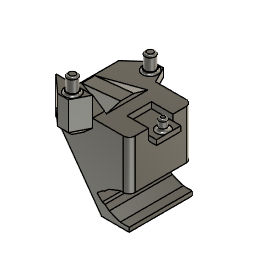
whiteboard v7 (Autodesk Fusion 360 archive; units mm, degrees)
design "Centre_pulley_mount"
Autodesk Fusion 360 part; units mm, degrees
sketch "Sketch1" plane through (0, 0, 0) normal (0, 1, 0) x (1, 0, 0)
  line L0 (36.78, 0) -> (0, 0)
  line L1 (0, 0) -> (0, -40.3)
  line L2 (0, -40.3) -> (6.2098, -40.3)
  line L3 (15.9457, -40.3) -> (36.78, -40.3)
  line L4 (18.4769, -2.1208) -> (18.4964, -2.1208)
  line L5 (36.78, -40.3) -> (36.78, -15.7708)
  line L6 (36.78, -2.0947) -> (36.78, 0)
  line L7 (6.2098, -40.3) -> (15.9457, -40.3)
  line L8 (26.7841, -13.675) -> (24.3642, -11.6584)
  line L9 (32.31, -15.7708) -> (26.7841, -13.675)
  line L10 (36.78, -15.7708) -> (32.31, -15.7708)
  line L11 (36.7605, -2.1208) -> (32.2906, -2.1335)
  line L12 (32.2906, -2.1335) -> (26.7706, -4.2451)
  line L13 (26.7706, -4.2451) -> (24.643, -6.0284)
  line L14 (36.7605, -2.1208) -> (36.78, -2.1208)
  line L15 (36.78, -2.1208) -> (36.78, -2.0947)
  line L16 (24.3642, -11.6584) -> (23.2561, -11.1913)
  line L17 (23.2561, -11.1913) -> (20.661, -9.0288)
  line L18 (24.643, -6.0284) -> (23.3467, -6.4358)
  line L19 (23.3467, -6.4358) -> (20.661, -9.0288)
  point P0 (18.4964, -8.9458)
  point P1 (18.4964, -8.9458)
  point P2 (36.6848, -8.6861)
  point P3 (36.6848, -8.6861)
  point P4 (36.78, -8.9458)
  point P5 (36.78, -8.9458)
  dimension "d19" = 40.3
  dimension "d21" = 36.78
  dimension "d31" = 13.65
  dimension "d32" = 4.47
  dimension "d33" = 159.23
  dimension "d34" = 160.964
  dimension "d36" = 5.91
  dimension "d37" = 3.15
  constraint horizontal L2
  constraint vertical L5
  constraint horizontal L0
  constraint vertical L1
  constraint collinear L2 L3
  constraint coincident P1 P0
  constraint coincident L0.end L1.start
  constraint collinear L5 L6
  constraint coincident L4 L6.start
  constraint parallel L3 L7
  constraint coincident P3 P2
  constraint coincident P5 P4
  constraint coincident L5.end L10.start
  constraint parallel L6 L15
  constraint parallel L8 L17
  measures "d19" distance of L1.end L0.end
  measures "d21" distance of L1 L5
  measures "d31" distance of L14.end L5.end
  measures "d32" distance of L9.start L5.end
  measures "d33" angle of L9 L10
  measures "d34" angle of L8 L9
  measures "d36" distance of L8.start L9.start
  measures "d37" distance of L8.start L8.end
extrude "Extrude1" add sketch "Sketch1" along normal blind 31.6
sketch "Sketch2" plane through (0, 0, 40.3) normal (0, 0, 1) x (-1, 0, 0)
  line L0 (0, 0) -> (-36.78, 0)
  line L1 (-36.78, 0) -> (-36.78, -31.6)
  line L2 (-36.78, -31.6) -> (0, -31.6)
  line L3 (0, -31.6) -> (0, 0)
  line L4 (-26, -21.9) -> (-36.78, -21.9)
  line L5 (-36.78, -21.9) -> (-36.78, -9.7)
  line L6 (-36.78, -9.7) -> (-26, -9.7)
  line L7 (-26, -9.7) -> (-26, -21.9)
  point P0 (-36.78, -15.8)
  point P1 (-36.78, -15.8)
  dimension "d42" = 12.2
  dimension "d43" = 10.78
  constraint horizontal L4
  constraint vertical L5
  constraint horizontal L6
  constraint vertical L7
  constraint coincident L1 L5.end
  constraint midpoint L5 P1
  constraint midpoint L1 P1
  constraint coincident P1 P0
  measures "d42" distance of L4.start L6.end
  measures "d43" distance of L4.start L4.end
extrude "Extrude2" cut sketch "Sketch2" against normal blind 2.5 contours L1 L4 L5 L6 L7
sketch "Sketch3" plane through (36.78, 0, 0) normal (1, 0, 0) x (0, 1, 0)
  line L0 (9.7, 37.8) -> (9.7, 40.3)
  line L1 (9.7, 40.3) -> (0, 40.3)
  line L2 (0, 40.3) -> (0, 15.7708)
  line L3 (0, 15.7708) -> (31.6, 15.7708)
  line L4 (31.6, 15.7708) -> (31.6, 40.3)
  line L5 (31.6, 40.3) -> (21.9, 40.3)
  line L6 (21.9, 40.3) -> (21.9, 37.8)
  line L7 (21.9, 37.8) -> (9.7, 37.8)
  line L8 (9.7, 37.8) -> (21.9, 37.8)
  line L9 (21.9, 37.8) -> (21.9, 35.8)
  line L10 (21.9, 35.8) -> (9.7, 35.8)
  line L11 (9.7, 35.8) -> (9.7, 37.8)
  dimension "d46" = 2
  constraint horizontal L8
  constraint vertical L9
  constraint horizontal L10
  constraint vertical L11
  constraint coincident L0.start L7.end
  constraint collinear L6 L9
  measures "d46" distance of L0.start L10.end
extrude "Extrude3" add sketch "Sketch3" along normal blind 3 contours L7 L8 L9 L10 L11
sketch "Sketch4" plane through (0, 0, 37.8) normal (0, 0, 1) x (-1, 0, 0)
  line L0 (-26, -9.7) -> (-36.78, -9.7)
  line L1 (-36.78, -9.7) -> (-39.78, -9.7)
  line L2 (-39.78, -9.7) -> (-39.78, -21.9)
  line L3 (-39.78, -21.9) -> (-36.78, -21.9)
  line L4 (-36.78, -21.9) -> (-26, -21.9)
  line L5 (-26, -21.9) -> (-26, -9.7)
  circle A0 centre (-37.9, -15.8) radius 1.9
  point P0 (-39.78, -15.8)
  dimension "d49" = 3.8
  dimension "d50" = 11.9
  constraint midpoint L2 P0
  constraint horizontal A0.centre P0
  measures "d49" diameter of A0
  measures "d50" distance of L5 A0.centre
extrude "Extrude4" add 1 faces at (39.78, 13.7667, 36.4667) along direction (1, 0, 0) blind 0.5
extrude "Extrude5" add sketch "Sketch4" along normal blind 5 contours L2 A0 | L2 A0
sketch "Sketch5" plane through (0, 0, 0) normal (0, -1, 0) x (1, 0, 0)
  line L0 (36.78, 2.1208) -> (36.7605, 2.1208)
  line L1 (36.7605, 2.1208) -> (32.2906, 2.1335)
  line L2 (32.2906, 2.1335) -> (26.7706, 4.2451)
  line L3 (26.7706, 4.2451) -> (24.643, 6.0284)
  line L4 (24.3642, 11.6584) -> (26.7841, 13.675)
  line L5 (26.7841, 13.675) -> (32.31, 15.7708)
  line L6 (32.31, 15.7708) -> (36.78, 15.7708)
  line L7 (36.78, 15.7708) -> (36.78, 40.3)
  line L8 (36.78, 40.3) -> (0, 40.3)
  line L9 (0, 40.3) -> (0, 0)
  line L10 (0, 0) -> (36.78, 0)
  line L11 (36.78, 0) -> (36.78, 2.1208)
  line L12 (0, 40.3) -> (18.39, 40.3)
  line L13 (18.39, 40.3) -> (18.39, 27.8397)
  line L14 (18.39, 27.8397) -> (0, 27.8397)
  line L15 (0, 27.8397) -> (0, 40.3)
  line L16 (24.643, 6.0284) -> (23.3467, 6.4358)
  line L17 (23.3467, 6.4358) -> (20.661, 9.0288)
  line L18 (20.661, 9.0288) -> (23.2561, 11.1913)
  line L19 (23.2561, 11.1913) -> (24.3642, 11.6584)
  point P0 (18.39, 40.3)
  constraint horizontal L12
  constraint vertical L13
  constraint horizontal L14
  constraint vertical L15
  constraint coincident L8.end L9.start
  constraint midpoint L8 P0
  constraint coincident P0 L12.end
extrude "Extrude6" add sketch "Sketch5" along normal blind 10 contours L8 L9 L12 L13 L14 L15
sketch "Sketch6" plane through (0, 0, 40.3) normal (0, 0, 1) x (-1, 0, 0)
  line L0 (-36.78, -9.7) -> (-26, -9.7)
  line L1 (-26, -9.7) -> (-26, -21.9)
  line L2 (-26, -21.9) -> (-36.78, -21.9)
  line L3 (-36.78, -21.9) -> (-36.78, -31.6)
  line L4 (-36.78, -31.6) -> (0, -31.6)
  line L5 (0, -31.6) -> (0, 10)
  line L6 (0, 10) -> (-18.39, 10)
  line L7 (-18.39, 10) -> (-18.39, 0)
  line L8 (-18.39, 0) -> (-36.78, 0)
  line L9 (-36.78, 0) -> (-36.78, -9.7)
  circle A0 centre (-12, 3.7) radius 2.5
  line L10 (-26, -15.8) -> (0, -15.8) construction
  circle A1 centre (-12, -35.3) radius 2.5
  dimension "d57" = 5
  dimension "d58" = 12
  dimension "d59" = 19.5
  dimension "d69" = 5
  constraint midpoint L1 L10.start
  constraint coincident L5 L10.end
  constraint perpendicular L5 L10
  constraint symmetric A0 L10 A1
  measures "d57" diameter of A0
  measures "d58" distance of L5 A0.centre
  measures "d59" distance of A0.centre L10
  measures "d69" diameter of A1
extrude "Extrude7" cut 1 faces at (6.13, -10, 36.1466) along direction (0, 1, 0) blind 2
chamfer "Chamfer1" distance 8 distance2 4 1 edges at (18.39, -8, 34.0698) measured on face at (18.39, -2.6667, 36.1466)
chamfer "Chamfer2" distance 8 distance2 9 1 edges at (0, -8, 34.0698) measured on face at (0, 21.0667, 22.7132)
chamfer "Chamfer3" distance 4 distance2 4 3 edges at (4.5, -4, 27.8397) (11.695, -8, 27.8397) (16.39, -4, 27.8397) measured on face at (6, -5.3333, 36.1466) measured on face at (9.13, -2.6667, 27.8397) measured on face at (17.0569, -2.6677, 36.1466)
sketch "Sketch7" plane through (0, 31.6, 0) normal (0, 1, 0) x (-1, 0, 0)
  line L0 (-36.7605, 2.1208) -> (-36.78, 2.1208)
  line L1 (-36.78, 2.1208) -> (-36.78, 0)
  line L2 (-36.78, 0) -> (0, 0)
  line L3 (0, 0) -> (0, 40.3)
  line L4 (0, 40.3) -> (-36.78, 40.3)
  line L5 (-36.78, 40.3) -> (-36.78, 15.7708)
  line L6 (-36.78, 15.7708) -> (-32.31, 15.7708)
  line L7 (-32.31, 15.7708) -> (-26.7841, 13.675)
  line L8 (-26.7841, 13.675) -> (-24.3642, 11.6584)
  line L9 (-24.643, 6.0284) -> (-26.7706, 4.2451)
  line L10 (-26.7706, 4.2451) -> (-32.2906, 2.1335)
  line L11 (-32.2906, 2.1335) -> (-36.7605, 2.1208)
  line L12 (0, 40.3) -> (-18.39, 40.3)
  line L13 (-18.39, 40.3) -> (-18.39, 32.3)
  line L14 (-18.39, 32.3) -> (0, 32.3)
  line L15 (0, 32.3) -> (0, 40.3)
  line L16 (-24.3642, 11.6584) -> (-23.2561, 11.1913)
  line L17 (-23.2561, 11.1913) -> (-20.661, 9.0288)
  line L18 (-20.661, 9.0288) -> (-23.3467, 6.4358)
  line L19 (-23.3467, 6.4358) -> (-24.643, 6.0284)
  point P0 (-18.39, 40.3)
  dimension "d68" = 8
  constraint horizontal L12
  constraint vertical L13
  constraint horizontal L14
  constraint vertical L15
  constraint coincident L3.end L4.start
  constraint midpoint L4 P0
  constraint coincident P0 L12.end
  measures "d68" distance of P0 L13.end
extrude "Extrude8" add sketch "Sketch7" along normal blind 8 contours L3 L4 L12 L13 L14 L15
chamfer "Chamfer4" distance 4 distance2 8 1 edges at (18.39, 39.6, 36.3) measured on face at (12.26, 39.6, 37.6333)
chamfer "Chamfer5" distance 9 distance2 8 1 edges at (0, 39.6, 36.3) measured on face at (4.7969, 39.6, 34.9667)
chamfer "Chamfer6" distance 4 distance2 4 3 edges at (11.695, 39.6, 32.3) (4.5, 35.6, 32.3) (16.39, 35.6, 32.3) measured on face at (12.5939, 39.6, 34.9667) measured on face at (6, 36.9333, 37.6333) measured on face at (17.0569, 34.2677, 37.6333)
extrude "Extrude9" add sketch "Sketch6" along normal blind 8 contours A0 | A1
sketch "Sketch8" plane through (0, 0, 40.3) normal (0, 0, 1) x (-1, 0, 0)
  circle A0 centre (-12, -35.3) radius 2.5
  circle A1 centre (-12, 3.7) radius 2.5
  line L0 (-9, -39.6) -> (0, -31.6)
  line L1 (0, -31.6) -> (0, 0)
  line L2 (0, 0) -> (-9, 8)
  line L3 (-9, 8) -> (-14.39, 8)
  line L4 (-14.39, 8) -> (-18.39, 0)
  line L5 (-18.39, 0) -> (-36.78, 0)
  line L6 (-36.78, 0) -> (-36.78, -9.7)
  line L7 (-36.78, -9.7) -> (-26, -9.7)
  line L8 (-26, -9.7) -> (-26, -21.9)
  line L9 (-26, -21.9) -> (-36.78, -21.9)
  line L10 (-36.78, -21.9) -> (-36.78, -31.6)
  line L11 (-36.78, -31.6) -> (-18.39, -31.6)
  line L12 (-18.39, -31.6) -> (-14.39, -39.6)
  line L13 (-14.39, -39.6) -> (-9, -39.6)
  circle A2 centre (-12, -35.3) radius 2.5
  circle A3 centre (-12, -35.3) radius 2.875
  dimension "d80" = 5.75
  constraint concentric A0 A2
  constraint concentric A2 A3
  measures "d80" diameter of A3
extrude "Extrude10" add sketch "Sketch8" along normal blind 1 contours A3
chamfer "Chamfer7" distance 23 distance2 32 1 edges at (0, 15.8, 0) measured on face at (24.52, 21.0667, 0)
fillet "Fillet1" radius 3 1 edges at (36.78, 0, 28.0354)
fillet "Fillet2" radius 3 1 edges at (36.78, 31.6, 28.0354)
fillet "Fillet3" radius 1 1 edges at (14.3308, 36.204, 48.3)
fillet "Fillet4" radius 1 1 edges at (39.6714, 16.4871, 42.8)
sketch "Sketch9" plane through (0, 0, 40.3) normal (0, 0, 1) x (-1, 0, 0)
  circle A0 centre (-12, -35.3) radius 2.875
  circle A1 centre (-12, 3.7) radius 2.5
  arc A2 (-36.78, -28.6) -> (-33.78, -31.6) centre (-33.78, -28.6) ccw
  line L0 (-33.78, -31.6) -> (-18.39, -31.6)
  line L1 (-18.39, -31.6) -> (-14.39, -39.6)
  line L2 (-14.39, -39.6) -> (-9, -39.6)
  line L3 (-9, -39.6) -> (0, -31.6)
  line L4 (0, -31.6) -> (0, 0)
  line L5 (0, 0) -> (-9, 8)
  line L6 (-9, 8) -> (-14.39, 8)
  line L7 (-14.39, 8) -> (-18.39, 0)
  line L8 (-18.39, 0) -> (-33.78, 0)
  arc A3 (-33.78, 0) -> (-36.78, -3) centre (-33.78, -3) ccw
  line L9 (-36.78, -3) -> (-36.78, -9.7)
  line L10 (-36.78, -9.7) -> (-26, -9.7)
  line L11 (-26, -9.7) -> (-26, -21.9)
  line L12 (-26, -21.9) -> (-36.78, -21.9)
  line L13 (-36.78, -21.9) -> (-36.78, -28.6)
  circle A4 centre (-12, 3.7) radius 2.5
  circle A5 centre (-12, 3.7) radius 2.875
  dimension "d93" = 5.75
  constraint concentric A1 A4
  constraint concentric A4 A5
  measures "d93" diameter of A5
extrude "Extrude11" add sketch "Sketch9" along normal blind 11 contours A5
extrude "Extrude12" add 1 faces at (11.2086, -2.7962, 48.3) along direction (0, 0, 1) blind 11
extrude "Extrude13" cut 1 faces at (11.2086, -2.7962, 59.3) along direction (0, 0, -1) blind 1
fillet "Fillet5" radius 1 1 edges at (14.3308, -4.604, 58.3)
sketch "Sketch10" plane through (0, 0, 0) normal (-1, 0, 0) x (0, -1, 0)
  line L0 (-31.6, 32) -> (0, 32)
  line L1 (0, 32) -> (0, 40.3)
  line L2 (0, 40.3) -> (-31.6, 40.3)
  line L3 (-31.6, 40.3) -> (-31.6, 36.3)
  line L4 (-31.6, 36.3) -> (-31.6, 32)
  line L5 (0, 32) -> (8.3989, 32)
  line L6 (8.3989, 32) -> (8.3989, 27.6433)
  line L7 (8.3989, 27.6433) -> (0, 27.6433)
  line L8 (0, 27.6433) -> (0, 32)
  constraint horizontal L5
  constraint vertical L6
  constraint horizontal L7
  constraint vertical L8
  constraint coincident L0.end L1.start
extrude "Extrude14" cut sketch "Sketch10" against normal blind 22 contours L5 L6 L7 L8
chamfer "Chamfer8" distance 4 distance2 4 3 edges at (4.5, -4, 32) (11.695, -8, 32) (16.39, -4, 32) measured on face at (3, -2.6667, 37.5333) measured on face at (12.5939, -8, 34.7667) measured on face at (15.7239, -5.3339, 37.5333)
sketch "Sketch11" plane through (0, 0, 40.3) normal (0, 0, 1) x (-1, 0, 0)
  circle A0 centre (-12, -35.3) radius 2.875
  circle A1 centre (-12, 3.7) radius 2.875
  line L0 (-0.5, -26.1) -> (-20, -26.1)
  line L1 (-20, -26.1) -> (-20, -5.5)
  line L2 (-20, -5.5) -> (-0.5, -5.5)
  line L3 (-0.5, -5.5) -> (-0.5, -26.1)
  line L4 (-26, -10.2) -> (-26, -21.9)
  arc A2 (-36.78, -28.6) -> (-33.78, -31.6) centre (-33.78, -28.6) ccw
  line L5 (-33.78, -31.6) -> (-18.39, -31.6)
  line L6 (-18.39, -31.6) -> (-14.39, -39.6)
  line L7 (-14.39, -39.6) -> (-9, -39.6)
  line L8 (-9, -39.6) -> (0, -31.6)
  line L9 (0, -31.6) -> (0, 0)
  line L10 (0, 0) -> (-9, 8)
  line L11 (-9, 8) -> (-14.39, 8)
  line L12 (-14.39, 8) -> (-18.39, 0)
  line L13 (-18.39, 0) -> (-33.78, 0)
  arc A3 (-33.78, 0) -> (-36.78, -3) centre (-33.78, -3) ccw
  line L14 (-36.78, -3) -> (-36.78, -9.7)
  line L15 (-36.78, -9.7) -> (-26, -9.7)
  line L16 (-26, -9.7) -> (-26, -21.9)
  line L17 (-26, -21.9) -> (-36.78, -21.9)
  line L18 (-36.78, -21.9) -> (-36.78, -28.6)
  point P0 (-0.5, -15.8)
  point P1 (-0.5, -15.8)
  dimension "d108" = 6
  dimension "d109" = 20.6
  constraint horizontal L0
  constraint vertical L1
  constraint horizontal L2
  constraint vertical L3
  constraint midpoint L3 P1
  constraint coincident P1 P0
  measures "d108" distance of L1 L4
  measures "d109" distance of L0.end L1.end
extrude "Extrude15" add sketch "Sketch11" along normal blind 2 contours L0 L1 L2 L3
chamfer "Chamfer11" distance 19.5 distance2 2 1 edges at (0.5, 15.8, 42.3) measured on face at (7, 12.3667, 42.3)
extrude "Extrude16" add 1 faces at (39.1133, 17.8333, 35.8) along direction (0, 0, -1) blind 1
extrude "Extrude17" cut 1 faces at (29.3333, 15.8, 37.8) along direction (0, 0, -1) blind 0.5
extrude "Extrude18" add 1 faces at (40.28, 13.7667, 35.6333) along direction (1, 0, 0) blind 0.5
fillet "Fillet8" radius 1.5 1 edges at (39.6714, 16.4871, 37.3)
chamfer "Chamfer13" distance 7 distance2 1.989 2 edges at (10.25, 26.1, 41.3) (10.25, 5.5, 41.3) measured on face at (6.9987, 12.3667, 40.9669) measured on face at (6.9987, 12.3667, 40.9669)
sketch "Sketch13" plane through (0, 0, 40.3) normal (0, 0, 1) x (-1, 0, 0)
  line L0 (-0.5, -12.5) -> (-0.5, -19.1)
  line L1 (-0.5, -19.1) -> (-19.9945, -26.1)
  line L2 (-19.9945, -26.1) -> (-20, -26.1)
  line L3 (-20, -26.1) -> (-20, -5.5)
  line L4 (-20, -5.5) -> (-19.9945, -5.5)
  line L5 (-19.9945, -5.5) -> (-0.5, -12.5)
  circle A0 centre (-12, 3.7) radius 2.875
  circle A1 centre (-12, -35.3) radius 2.875
  arc A2 (-36.78, -28.6) -> (-33.78, -31.6) centre (-33.78, -28.6) ccw
  line L6 (-33.78, -31.6) -> (-18.39, -31.6)
  line L7 (-18.39, -31.6) -> (-14.39, -39.6)
  line L8 (-14.39, -39.6) -> (-9, -39.6)
  line L9 (-9, -39.6) -> (0, -31.6)
  line L10 (0, -31.6) -> (0, 0)
  line L11 (0, 0) -> (-9, 8)
  line L12 (-9, 8) -> (-14.39, 8)
  line L13 (-14.39, 8) -> (-18.39, 0)
  line L14 (-18.39, 0) -> (-33.78, 0)
  arc A3 (-33.78, 0) -> (-36.78, -3) centre (-33.78, -3) ccw
  line L15 (-36.78, -3) -> (-36.78, -9.7)
  line L16 (-36.78, -9.7) -> (-26, -9.7)
  line L17 (-26, -9.7) -> (-26, -21.9)
  line L18 (-26, -21.9) -> (-36.78, -21.9)
  line L19 (-36.78, -21.9) -> (-36.78, -28.6)
  circle A4 centre (-12, 3.7) radius 2.875
  line L20 (0, 0) -> (-9, 8)
  line L21 (-9, 8) -> (-14.39, 8)
  line L22 (-14.39, 8) -> (-18.39, 0)
  line L23 (-18.39, -6.0761) -> (0, -6.0761)
  line L24 (0, -6.0761) -> (0, 0)
  line L25 (-18.39, -6.0761) -> (-18.39, 0)
  circle A5 centre (-12, -35.3) radius 2.875
  line L26 (0, -31.6) -> (-9, -39.6)
  line L27 (-9, -39.6) -> (-14.39, -39.6)
  line L28 (-14.39, -39.6) -> (-18.39, -31.6)
  line L29 (-18.39, -31.6) -> (-18.39, -25.5239)
  line L30 (-18.39, -25.5239) -> (0, -25.5239)
  line L31 (0, -25.5239) -> (0, -31.6)
  constraint concentric A0 A4
  constraint coincident L10.end L11.start
  constraint coincident L11.end L12.start
  constraint coincident L12.end L13.start
  constraint coincident L13.end L14.start
  constraint coincident L5 L23.start
  constraint coincident L10 L23.end
  constraint perpendicular L10 L23
  constraint perpendicular L14 L25
  constraint concentric A1 A5
  constraint coincident L9.end L10.start
  constraint coincident L8.end L9.start
  constraint coincident L7.end L8.start
  constraint coincident L6.end L7.start
  constraint coincident L1 L29.end
  constraint perpendicular L6 L29
  constraint coincident L10 L30.end
  constraint perpendicular L10 L30
extrude "Extrude19" add sketch "Sketch13" along normal blind 10 contours L10 L11 L12 L13 L20 L21 L22 L23 L24 L25
chamfer "Chamfer14" distance 6 distance2 10 1 edges at (9.195, 6.0761, 50.3) measured on face at (10.0145, 3.7688, 50.3)
fillet "Fillet9" radius 1 1 edges at (14.6804, -2.6604, 50.3)
fillet "Fillet10" radius 1 1 edges at (14.6804, 34.2604, 40.3)

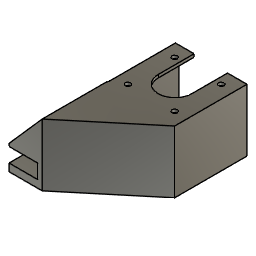
design "motor_mount_top_right"
Autodesk Fusion 360 part; units mm, degrees
sketch "Sketch1" plane through (0, 0, 0) normal (0, 0, 1) x (1, 0, 0)
  line L0 (0, 20) -> (22, 20)
  line L1 (22, -20) -> (0, -20)
  line L2 (0, -20) -> (0, 20)
  line L3 (22, 68) -> (70, 68)
  line L4 (70, 68) -> (70, 20)
  line L5 (22, 20) -> (22, 68)
  line L6 (22, -20) -> (70, 20)
  dimension "d1" = 22
  dimension "d2" = 48
  dimension "d3" = 48
  dimension "d4" = 40
  dimension "d5" = 22
  dimension "d6" = 48
  constraint horizontal L0
  constraint horizontal L1
  constraint vertical L2
  constraint horizontal L3
  constraint vertical L4
  constraint vertical L5
  constraint midpoint L2 origin
  measures "d1" distance of L0.start L0.end
  measures "d2" distance of L0.end L3.start
  measures "d3" distance of L3.start L3.end
  measures "d4" distance of L0.start L1.end
  measures "d5" distance of L1.end L1.start
  measures "d6" distance of L3.end L4.end
extrude "Extrude1" add sketch "Sketch1" along normal blind 2
sketch "Sketch2" plane through (0, 0, 2) normal (0, 0, 1) x (-1, 0, 0)
  line L0 (0, 20) -> (-22, 20)
  line L1 (-22, 20) -> (-70, -20)
  line L2 (-70, -20) -> (-70, -68)
  line L3 (-70, -68) -> (-22, -68)
  line L4 (-22, -68) -> (-22, -20)
  line L5 (-22, -20) -> (0, -20)
  line L6 (0, -20) -> (0, 20)
  line L7 (-28.8, -65.2) -> (-63.2, -65.2)
  line L8 (-67.2, -61.2) -> (-67.2, -26.8)
  line L9 (-63.2, -22.8) -> (-28.8, -22.8)
  line L10 (-24.8, -26.8) -> (-24.8, -61.2)
  line L11 (-28.8, -65.2) -> (-24.8, -61.2)
  line L12 (-28.8, -22.8) -> (-24.8, -26.8)
  line L13 (-67.2, -26.8) -> (-63.2, -22.8)
  line L14 (-63.2, -65.2) -> (-67.2, -61.2)
  point P0 (-24.8, -65.2)
  point P1 (-67.2, -65.2)
  point P2 (-67.2, -22.8)
  point P3 (-24.8, -22.8)
  point P4 (-46, -68)
  point P5 (-46, -65.2)
  point P6 (-22, -44)
  point P7 (-24.8, -44)
  dimension "d9" = 42.4
  dimension "d10" = 42.4
  dimension "d11" = 4
  dimension "d12" = 4
  dimension "d13" = 4
  dimension "d14" = 4
  dimension "d15" = 4
  dimension "d16" = 4
  dimension "d17" = 4
  dimension "d18" = 4
  constraint horizontal L7
  constraint vertical L8
  constraint horizontal L9
  constraint vertical L10
  constraint midpoint L3 P4
  constraint vertical P4 P5
  constraint midpoint L4 P6
  constraint horizontal P6 P7
  constraint coincident L7 P5
  constraint coincident L10 P7
  constraint coincident P0 L7
  constraint coincident P0 L10
  constraint coincident P3 L9
  constraint coincident P3 L10
  constraint coincident P2 L8
  constraint coincident P2 L9
  constraint coincident P1 L7
  constraint coincident P1 L8
  measures "d9" distance of P0 P1
  measures "d10" distance of P0 P3
  measures "d11" distance of P0 L7.start
  measures "d12" distance of P0 L10.end
  measures "d13" distance of P3 L9.end
  measures "d14" distance of P3 L10.start
  measures "d15" distance of P2 L8.end
  measures "d16" distance of P2 L9.start
  measures "d17" distance of P1 L7.end
  measures "d18" distance of P1 L8.start
extrude "Extrude2" add sketch "Sketch2" along normal blind 33.8
sketch "Sketch3" plane through (0, 0, 35.8) normal (0, 0, 1) x (-1, 0, 0)
  line L0 (-24.8, -61.2) -> (-28.8, -65.2)
  line L1 (-28.8, -65.2) -> (-63.2, -65.2)
  line L2 (-63.2, -65.2) -> (-67.2, -61.2)
  line L3 (-67.2, -61.2) -> (-67.2, -26.8)
  line L4 (-67.2, -26.8) -> (-63.2, -22.8)
  line L5 (-63.2, -22.8) -> (-28.8, -22.8)
  line L6 (-28.8, -22.8) -> (-24.8, -26.8)
  line L7 (-24.8, -26.8) -> (-24.8, -61.2)
  line L8 (0, -20) -> (0, 20)
  line L9 (0, 20) -> (-22, 20)
  line L10 (-22, 20) -> (-70, -20)
  line L11 (-70, -20) -> (-70, -68)
  line L12 (-70, -68) -> (-22, -68)
  line L13 (-22, -68) -> (-22, -20)
  line L14 (-22, -20) -> (0, -20)
  line L15 (-22, -68) -> (-22, -20)
  line L16 (-22, -20) -> (0, -20)
  line L17 (0, -20) -> (0, 20)
  line L18 (0, 20) -> (-22, 20)
  line L19 (-22, 20) -> (-70, -20)
  line L20 (-70, -20) -> (-70, -68)
  line L21 (-57.1, -68) -> (-57.1, -44.2)
  line L22 (-34.9, -44.2) -> (-34.9, -68)
  arc A0 (-34.9, -44.2) -> (-57.1, -44.2) centre (-46, -44.2) ccw
  line L23 (-70, -68) -> (-57.1, -68)
  line L24 (-34.9, -68) -> (-22, -68)
  line L25 (-61.5, -28.5) -> (-30.5, -28.5) construction
  line L26 (-30.5, -28.5) -> (-30.5, -59.5) construction
  line L27 (-30.5, -59.5) -> (-61.5, -59.5) construction
  line L28 (-61.5, -59.5) -> (-61.5, -28.5) construction
  circle A1 centre (-30.5, -28.5) radius 1.75
  circle A2 centre (-30.5, -59.5) radius 1.75
  circle A3 centre (-61.5, -28.5) radius 1.75
  circle A4 centre (-61.5, -59.5) radius 1.75
  point P0 (-46, -68)
  point P1 (-46, -68)
  point P2 (-46, -28.5)
  point P3 (-46, -22.8)
  point P4 (-30.5, -44)
  point P5 (-24.8, -44)
  dimension "d21" = 22.2
  dimension "d24" = 31
  dimension "d25" = 31
  dimension "d26" = 3.5
  dimension "d27" = 3.5
  dimension "d28" = 3.5
  dimension "d29" = 3.5
  constraint coincident L12.end L13.start
  constraint coincident L13.end L14.start
  constraint coincident L8.start L14.end
  constraint coincident L8.end L9.start
  constraint coincident L9.end L10.start
  constraint coincident L10.end L11.start
  constraint coincident L11.end L12.start
  constraint vertical L21
  constraint vertical L22
  constraint coincident L12 L22.end
  constraint midpoint L12 P1
  constraint coincident P1 P0
  constraint tangent L22 A0
  constraint collinear L23 L24
  constraint horizontal L25
  constraint vertical L26
  constraint horizontal L27
  constraint vertical L28
  constraint midpoint L25 P2
  constraint midpoint L5 P3
  constraint vertical P2 P3
  constraint midpoint L26 P4
  constraint midpoint L7 P5
  constraint horizontal P4 P5
  constraint coincident L25.end L26.start
  constraint coincident L26.end L27.start
  constraint coincident L25.start L28.end
  constraint coincident L27.end L28.start
  measures "d21" distance of L21.end L22.start
  measures "d24" distance of L25.start L25.end
  measures "d25" distance of L25.start L27.end
  measures "d26" diameter of A1
  measures "d27" diameter of A2
  measures "d28" diameter of A3
  measures "d29" diameter of A4
extrude "Extrude3" add sketch "Sketch3" along normal blind 2 contours L0 L1 L2 L3 L4 L5 L6 L7 L8 L9 L10 L11 L12 L13 L14 L15 L16 L17 L18 L19 L20 L21 L22 L23 L24 | L0 L1 L2 L3 L4 L5 L6 L7 L21 L22 A0
sketch "Sketch4" plane through (0, 68, 0) normal (0, 1, 0) x (-1, 0, 0)
  line L0 (-70, 0) -> (-22, 0)
  line L1 (-22, 0) -> (-22, 37.8)
  line L2 (-22, 37.8) -> (-34.9, 37.8)
  line L3 (-34.9, 37.8) -> (-34.9, 35.8)
  line L4 (-34.9, 35.8) -> (-57.1, 35.8)
  line L5 (-57.1, 35.8) -> (-70, 35.8)
  line L6 (-70, 35.8) -> (-70, 0)
  line L7 (-67.2, 35.8) -> (-24.8, 35.8)
  line L8 (-24.8, 35.8) -> (-24.8, 2)
  line L9 (-24.8, 2) -> (-67.2, 2)
  line L10 (-67.2, 2) -> (-67.2, 35.8)
  dimension "d32" = 2.8
  dimension "d33" = 2.8
  dimension "d34" = 2
  constraint horizontal L7
  constraint vertical L8
  constraint horizontal L9
  constraint vertical L10
  constraint coincident L5 L7.start
  measures "d32" distance of L6 L10
  measures "d33" distance of L1 L8
  measures "d34" distance of L0 L9
extrude "Extrude4" cut sketch "Sketch4" against normal blind 9 contours L4 L5 L7 L8 L9 L10
sketch "Sketch5" plane through (0, 0, 0) normal (-1, 0, 0) x (0, -1, 0)
  line L0 (-20, 0) -> (20, 0)
  line L1 (20, 0) -> (20, 37.8)
  line L2 (20, 37.8) -> (-20, 37.8)
  line L3 (-20, 37.8) -> (-20, 0)
  line L4 (-18, 2) -> (18, 2)
  line L5 (18, 2) -> (18, 11)
  line L6 (18, 11) -> (-18, 11)
  line L7 (-18, 11) -> (-18, 2)
  point P0 (0, 2)
  dimension "d37" = 36
  dimension "d38" = 9
  dimension "d39" = 2
  constraint horizontal L4
  constraint vertical L5
  constraint horizontal L6
  constraint vertical L7
  constraint midpoint L4 P0
  constraint vertical origin P0
  measures "d37" distance of L5.end L6.end
  measures "d38" distance of L4.start L6.end
  measures "d39" distance of L0 L4
extrude "Extrude5" cut sketch "Sketch5" against normal blind 19 contours L4 L5 L6 L7
fillet "Fillet1" radius 4.5 1 edges at (19, 18, 6.5)
sketch "Sketch6" plane through (0, 0, 0) normal (-1, 0, 0) x (0, -1, 0)
  line L0 (18, 2) -> (-18, 2)
  line L1 (-18, 2) -> (-18, 11)
  line L2 (-18, 11) -> (18, 11)
  line L3 (18, 11) -> (18, 2)
  line L4 (-20, 0) -> (20, 0)
  line L5 (20, 0) -> (20, 37.8)
  line L6 (20, 37.8) -> (-20, 37.8)
  line L7 (-20, 37.8) -> (-20, 0)
  line L8 (18, 11) -> (20, 11)
  line L9 (20, 11) -> (20, 2)
  line L10 (20, 2) -> (18, 2)
  line L11 (18, 2) -> (18, 11)
  constraint horizontal L8
  constraint vertical L9
  constraint horizontal L10
  constraint vertical L11
  constraint coincident L5 L9.end
  constraint coincident L2.end L3.start
extrude "Extrude6" cut sketch "Sketch6" against normal blind 19 contours L3 L5 L8 L9 L10 L11
chamfer "Chamfer1" distance 22 distance2 25 1 edges at (0, 0, 37.8) measured on face at (38, 11.323, 37.8)
fillet "Fillet2" radius 4.5 1 edges at (22, 20, 18.9)
sketch "Sketch7" plane through (0, 0, 37.8) normal (0, 0, 1) x (-1, 0, 0)
  line L0 (-22, -24.5) -> (-22, 20)
  line L1 (-22, 20) -> (-70, -20)
  line L2 (-70, -20) -> (-70, -68)
  line L3 (-70, -68) -> (-57.1, -68)
  line L4 (-57.1, -68) -> (-57.1, -44.2)
  arc A0 (-34.9, -44.2) -> (-57.1, -44.2) centre (-46, -44.2) ccw
  line L5 (-34.9, -44.2) -> (-34.9, -68)
  line L6 (-34.9, -68) -> (-22, -68)
  line L7 (-22, -68) -> (-22, -24.5)
  circle A1 centre (-30.5, -28.5) radius 1.75
  circle A2 centre (-61.5, -59.5) radius 1.75
  circle A3 centre (-61.5, -28.5) radius 1.75
  circle A4 centre (-30.5, -59.5) radius 1.75
  circle A5 centre (-26, -16) radius 2.5
  dimension "d50" = 5
  measures "d50" diameter of A5
fillet "Fillet3" radius 0.5 1 edges at (22, 46.25, 37.8)
sketch "Sketch8" plane through (0, 0, 2) normal (0, 0, 1) x (-1, 0, 0)
  line L0 (-19, 20) -> (-19, -13.5)
  arc A0 (-19, -13.5) -> (-14.5, -18) centre (-14.5, -13.5) ccw
  line L1 (-14.5, -18) -> (0, -18)
  line L2 (-17.682, -16.682) -> (-12.3791, -11.3782) construction
  circle A1 centre (-12.3791, -11.3782) radius 2
  line L3 (0, -18) -> (0, 20)
  line L4 (0, 20) -> (-19, 20)
  dimension "d61" = 7.5
  dimension "d62" = 4
  constraint midpoint A0 L2.start
  constraint coincident L2.end A1.centre
  measures "d61" distance of L2.start L2.end
  measures "d62" diameter of A1
extrude "Extrude8" cut sketch "Sketch8" along normal blind 29 contours A1
sketch "Sketch9" plane through (0, 0, 2) normal (0, 0, 1) x (-1, 0, 0)
  line L0 (-19, 20) -> (-19, -13.5)
  arc A0 (-19, -13.5) -> (-14.5, -18) centre (-14.5, -13.5) ccw
  line L1 (-14.5, -18) -> (0, -18)
  circle A1 centre (-12.3839, -11.3763) radius 2
  line L2 (0, -18) -> (0, 20)
  line L3 (0, 20) -> (-19, 20)
  dimension "d65" = 4
  measures "d65" diameter of A1
extrude "Extrude9" cut sketch "Sketch9" against normal blind 2 contours A1
sketch "Sketch10" plane through (0, 0, 37.8) normal (0, 0, 1) x (-1, 0, 0)
  line L0 (-57.1, -68) -> (-57.1, -44.2)
  arc A0 (-34.9, -44.2) -> (-57.1, -44.2) centre (-46, -44.2) ccw
  line L1 (-34.9, -44.2) -> (-34.9, -68)
  line L2 (-22, 20) -> (-70, -20)
  circle A1 centre (-30.5, -28.5) radius 1.75
  circle A2 centre (-61.5, -59.5) radius 1.75
  circle A3 centre (-61.5, -28.5) radius 1.75
  circle A4 centre (-30.5, -59.5) radius 1.75
  circle A5 centre (-12.3826, -11.3766) radius 4
  arc A6 (-22, -22.3206) -> (-22.5, -24.5) centre (-17.5, -24.5) ccw
  line L3 (-22, -22.3206) -> (-22, 20)
  line L4 (-70, -20) -> (-70, -68)
  line L5 (-70, -68) -> (-57.1, -68)
  line L6 (-34.9, -68) -> (-22.5, -68)
  line L7 (-22.5, -68) -> (-22.5, -24.5)
  dimension "d69" = 8
  measures "d69" diameter of A5
extrude "Extrude10" cut sketch "Sketch10" against normal blind 19 contours A5
extrude "Extrude11" add 1 faces at (15.6566, 10.8985, 18.8) along direction (0, 0, 1) blind 0.5
extrude "Extrude12" add 1 faces at (54, 37.5, 0) along direction (0, 0, -1) blind 4
extrude "Extrude13" cut 1 faces at (54, 37.5, -4) along direction (0, 0, 1) blind 1
sketch "Sketch11" plane through (0, 0, -3) normal (0, 0, -1) x (1, 0, 0)
  circle A0 centre (12.3839, -11.3763) radius 2
  line L0 (22, 20) -> (0, 20)
  line L1 (0, 20) -> (0, -20)
  line L2 (0, -20) -> (17.5, -20)
  arc A1 (22, -24.5) -> (17.5, -20) centre (17.5, -24.5) ccw
  line L3 (22, -24.5) -> (22, -68)
  line L4 (22, -68) -> (70, -68)
  line L5 (70, -68) -> (70, -20)
  line L6 (70, -20) -> (22, 20)
  circle A2 centre (12.3839, -11.3763) radius 4.25
  dimension "d78" = 8.5
  constraint concentric A0 A2
  measures "d78" diameter of A2
extrude "Extrude14" cut sketch "Sketch11" against normal blind 3.2 contours A2
extrude "Extrude15" cut 1 faces at (15.6566, 10.8985, 19.3) along direction (0, 0, -1) blind 2
extrude "Extrude16" add 1 faces at (54, 37.5, -3) along direction (0, 0, -1) blind 0.5
extrude "Extrude17" cut 1 faces at (15.6566, 10.8985, 17.3) along direction (0, 0, -1) blind 0.5
extrude "Extrude18" cut 1 faces at (10.381, -10.203, 2) along direction (0, 0, -1) blind 0.5
extrude "Extrude19" cut 1 faces at (40.2667, 48.4, 2) along direction (0, 0, -1) blind 1
equation "d5 = d1"
equation "d6 = d2"
equation "d10 = d9"
equation "d12 = d11"
equation "d14 = d13"
equation "d16 = d15"
equation "d18 = d17"
equation "d25 = d24"
equation "d33 = d32"

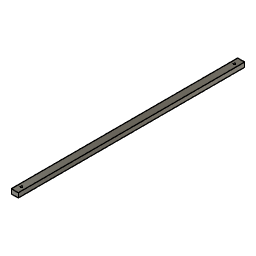
design "linear bar"
Autodesk Fusion 360 part; units mm, degrees
sketch "Sketch1" plane through (0, 0, 0) normal (0, 0, 1) x (1, 0, 0)
  line L0 (-6.13, 200) -> (6.13, 200)
  line L1 (6.13, 200) -> (6.13, -200)
  line L2 (6.13, -200) -> (-6.13, -200)
  line L3 (-6.13, -200) -> (-6.13, 200)
  circle A0 centre (0, 188.1) radius 1.9
  line L4 (-6.13, 0) -> (6.13, 0) construction
  circle A1 centre (0, -188.1) radius 1.9
  point P0 (0, 200)
  point P1 (-6.13, 0)
  dimension "d1" = 400
  dimension "d2" = 12.26
  dimension "d3" = 3.8
  dimension "d4" = 11.9
  constraint horizontal L0
  constraint vertical L1
  constraint horizontal L2
  constraint vertical L3
  constraint midpoint L0 P0
  constraint vertical origin P0
  constraint midpoint L3 P1
  constraint horizontal origin P1
  constraint vertical P0 A0.centre
  constraint coincident P1 L4.start
  constraint midpoint L1 L4.end
  constraint symmetric A0 L4 A1
  measures "d1" distance of L0.start L2.end
  measures "d2" distance of L0.start L0.end
  measures "d3" diameter of A0
  measures "d4" distance of P0 A0.centre
extrude "Extrude1" add sketch "Sketch1" along normal blind 8
